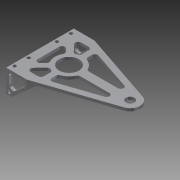
# Autodesk Inventor part: lower bix side plate 3.5
Saved by Autodesk Inventor 2012 (Build 160160000, 160)
## iProperties
Created: 2012-12-28
Part Number: lower bix side plate 3.5
Material: Default
Document SubType Name: Modeling
Designer: Bryce
Density: 1 g/cm^3
Author: Bryce
Autodesk Inventor part; units mm, degrees
ref_plane "YZ Plane" through (0, 0, 0) normal (1, 0, 0) x (0, 1, 0)
ref_plane "XZ Plane" through (0, 0, 0) normal (0, 1, 0) x (-1, 0, 0)
ref_plane "XY Plane" through (0, 0, 0) normal (0, 0, 1) x (1, 0, 0)
sketch "Sketch1" plane through (0, 0, 0) normal (0, 0, 1) x (1, 0, 0)
  line L0 (-34.925, 101.6) -> (34.925, 101.6)
  line L1 (34.925, 101.6) -> (34.925, 68.8594)
  line L2 (-34.925, 68.8594) -> (-34.925, 101.6)
  line L3 (-34.925, 68.8594) -> (-10.5309, -3.5479)
  line L4 (34.925, 68.8594) -> (10.5309, -3.5479)
  arc A0 (-10.5309, -3.5479) -> (10.5309, -3.5479) centre (0, 0) ccw
  circle A1 centre (0, 0) radius 4.7625
  circle A2 centre (0, 68.8594) radius 11.1125
  line L5 (0, 68.8594) -> (-34.925, 68.8594) construction
  line L6 (0, 68.8594) -> (34.925, 68.8594) construction
  line L7 (0, 68.8594) -> (-34.925, 101.6) construction
  line L8 (0, 68.8594) -> (34.925, 101.6) construction
  line L9 (0, 68.8594) -> (0, 0) construction
  line L10 (0, 68.8594) -> (0, 0) construction
  arc A3 (-15.5543, 65.6844) -> (-4.7625, 53.7156) centre (0, 68.8594) ccw
  arc A4 (4.7625, 53.7156) -> (15.5543, 65.6844) centre (0, 68.8594) ccw
  arc A5 (15.5543, 72.0344) -> (13.5191, 77.181) centre (0, 68.8594) ccw
  arc A6 (9.1762, 81.8137) -> (-9.1762, 81.8137) centre (0, 68.8594) ccw
  arc A7 (-13.5191, 77.181) -> (-15.5543, 72.0344) centre (0, 68.8594) ccw
  line L11 (-4.7625, 53.7156) -> (-4.7625, 10.0402)
  line L12 (4.7625, 53.7156) -> (4.7625, 10.0402)
  arc A8 (-4.7625, 10.0402) -> (-7.7188, 7.9942) centre (0, 0) ccw
  arc A9 (7.7188, 7.9942) -> (4.7625, 10.0402) centre (0, 0) ccw
  line L13 (-27.1547, 65.6844) -> (-7.7188, 7.9942)
  line L14 (7.7188, 7.9942) -> (27.1547, 65.6844)
  line L15 (-27.1547, 65.6844) -> (-15.5543, 65.6844)
  line L16 (-28.575, 72.0344) -> (-15.5543, 72.0344)
  line L17 (15.5543, 65.6844) -> (27.1547, 65.6844)
  line L18 (15.5543, 72.0344) -> (28.575, 72.0344)
  line L19 (-28.575, 91.2952) -> (-13.5191, 77.181)
  line L20 (-20.1222, 92.075) -> (-9.1762, 81.8137)
  line L21 (20.1222, 92.075) -> (9.1762, 81.8137)
  line L22 (28.575, 91.2952) -> (13.5191, 77.181)
  line L23 (-28.575, 91.2952) -> (-28.575, 72.0344)
  line L24 (-20.1222, 92.075) -> (20.1222, 92.075)
  line L25 (28.575, 91.2952) -> (28.575, 72.0344)
  arc A10 (4.7625, 18.588) -> (10.9463, 17.5744) centre (7.9375, 18.588) ccw
  arc A11 (-10.9463, 17.5744) -> (-4.7625, 18.588) centre (-7.9375, 18.588) ccw
  point P0 (-31.75, 98.425)
  point P1 (31.75, 98.425)
  point P2 (-15.875, 98.425)
  point P3 (15.875, 98.425)
  dimension "d0" = 69.85
  dimension "d1" = 101.6
  dimension "d2" = 34.925
  dimension "d6" = 18.619
  dimension "d7" = 9.525
  dimension "d8" = 32.7406
  dimension "d9" = 22.225
  dimension "d12" = 15.875
  dimension "d13" = 4.7625
  dimension "d14" = 4.7625
  dimension "d15" = 6.35
  dimension "d16" = 6.35
  dimension "d17" = 3.175
  dimension "d18" = 3.175
  dimension "d19" = 3.175
  dimension "d20" = 3.175
  dimension "d21" = 3.175
  dimension "d22" = 3.175
  dimension "d24" = 3.175
  dimension "d25" = 3.175
  dimension "d26" = 6.35
  dimension "d27" = 9.525
  dimension "d28" = 6.35
  dimension "d32" = 3.175
  dimension "d33" = 3.175
  dimension "d35" = 3.175
  dimension "d36" = 3.175
  dimension "d62" = 19.05
  dimension "d63" = 19.05
  dimension "d69" = 3.175
  dimension "d70" = 18.619
  dimension "d71" = 11.1125
  constraints: 52 end point, 20 point on circle, 13 parallel, 12 centre point, 9 coincident, 7 equal radius, 7 perpendicular, 5 tangent, 4 horizontal alignment, 4 point on line, 1 collinear, 1 horizontal, 1 vertical alignment
  measures "d0" distance between parallel lines of L1 L2
  measures "d1" distance from line of point (0, 0) L0
  measures "d2" distance from line of point (0, 0) L2
  measures "d6" angle of L1 L4
  measures "d7" diameter of A1
  measures "d8" distance from line of L5.start L0
  measures "d9" diameter of A2
  measures "d12" radius of A3
  measures "d13" distance between parallel lines of L9 L11
  measures "d14" distance between parallel lines of L9 L12
  measures "d15" distance between parallel lines of L3 L13
  measures "d16" distance between parallel lines of L4 L14
  measures "d17" distance between parallel lines of L15 L5
  measures "d18" distance between parallel lines of L5 L16
  measures "d19" distance between parallel lines of L17 L6
  measures "d20" distance between parallel lines of L6 L18
  measures "d21" distance between parallel lines of L8 L21
  measures "d22" distance between parallel lines of L8 L22
  measures "d24" distance between parallel lines of L7 L19
  measures "d25" distance between parallel lines of L7 L20
  measures "d26" distance between parallel lines of L23 L2
  measures "d27" distance between parallel lines of L0 L24
  measures "d28" distance between parallel lines of L1 L25
  measures "d32" distance from line of L2 point (-31.75, 98.425)
  measures "d33" distance from line of L0 point (-31.75, 98.425)
  measures "d35" distance from line of L0 point (31.75, 98.425)
  measures "d36" distance from line of L1 point (31.75, 98.425)
  measures "d62" distance from line of L2 point (-15.875, 98.425)
  measures "d63" distance from line of point (15.875, 98.425) L1
  measures "d69" radius of A11
  measures "d70" angle of L3 L2
  measures "d71" radius of A0
extrude "Extrusion1" add sketch "Sketch1" against normal blind 3.175 contours L0 L1 L4 A0 L3 L2 | A3 L11 A11 L13 L15 | L11 A8 L13 A11 | A4 L17 L14 A10 L12 | A10 L14 A9 L12 | A5 L22 L25 L18 | A6 L20 L24 L21 | A7 L16 L23 L19
extrude "Extrusion2" cut sketch "Sketch1" against normal blind 3.175 contours A3 L11 A11 L13 L15 | A4 L17 L14 A10 L12 | A5 L22 L25 L18 | A6 L20 L24 L21 | A7 L16 L23 L19
fillet "Fillet1" radius 3.175 16 edges at (-28.575, 72.0344, -1.5875) (-28.575, 91.2952, -1.5875) (28.575, 91.2952, -1.5875) (28.575, 72.0344, -1.5875) (15.5543, 72.0344, -1.5875) (13.5191, 77.181, -1.5875) (9.1762, 81.8137, -1.5875) (-9.1762, 81.8137, -1.5875) (-13.5191, 77.181, -1.5875) (-15.5543, 72.0344, -1.5875) (15.5543, 65.6844, -1.5875) (27.1547, 65.6844, -1.5875) (4.7625, 53.7156, -1.5875) (-4.7625, 53.7156, -1.5875) (-15.5543, 65.6844, -1.5875) (-27.1547, 65.6844, -1.5875)
hole "Hole1" at (-31.75, 98.425, 0) at (31.75, 98.425, 0) at (-15.875, 98.425, 0) at (15.875, 98.425, 0) direction (0, 0, -1) diameter 3.6576 end through all
sketch "Sketch2" plane through (0, 0, 0) normal (0, 0, 1) x (1, 0, 0)
  line L0 (-20.1222, 92.075) -> (20.1222, 92.075) projected
  circle A0 centre (0, 68.8594) radius 11.1125 projected
  line L1 (34.925, 68.8594) -> (10.5309, -3.5479) projected
  line L2 (34.925, 101.6) -> (34.925, 68.8594) projected
  circle A1 centre (15.875, 98.425) radius 1.8288 projected
  circle A2 centre (-15.875, 98.425) radius 1.8288 projected
  circle A3 centre (-15.875, 98.425) radius 1.8288
  circle A4 centre (15.875, 98.425) radius 1.8288
  line L3 (-10.9463, 17.5744) -> (-25.7435, 61.4957) projected
  line L4 (-34.925, 101.6) -> (34.925, 101.6) projected
  line L5 (-34.925, 68.8594) -> (-38.1, 78.2835)
  line L6 (-38.1, 78.2835) -> (-38.1, 101.6)
  line L7 (-34.925, 101.6) -> (-38.1, 101.6)
  line L8 (34.925, 101.6) -> (38.1, 101.6)
  line L9 (38.1, 101.6) -> (38.1, 78.2835)
  line L10 (38.1, 78.2835) -> (34.925, 68.8594)
  line L11 (-34.925, 101.6) -> (-34.925, 68.8594)
  line L12 (34.925, 101.6) -> (34.925, 68.8594)
  dimension "d53" = 22.225
  dimension "d75" = 3.175
  dimension "d76" = 3.175
  constraints: 16 end point, 4 parallel, 2 centre point, 2 coincident, 2 collinear, 2 concentric, 2 perpendicular
  measures "d53" diameter of A0
  measures "d75" distance of L2.start L8.end
  measures "d76" distance of L4.start L6.end
fillet "Fillet6" radius 3.175 2 edges at (-20.1222, 92.075, -1.5875) (20.1222, 92.075, -1.5875)
extrude "Extrusion7" add sketch "Sketch2" against normal blind 25.4 contours L8 L9 L10 L2 | L5 L6 L7 L11
sketch "Sketch4" plane through (-38.1, 78.2835, 0) normal (-1, 0, 0) x (0, 0, 1)
  line L0 (-25.4, 23.3165) -> (-25.4, 0) projected
  line L1 (0, 23.3165) -> (0, 0) projected
  line L2 (0, 23.3165) -> (-25.4, 23.3165) projected
  circle A0 centre (-22.225, 20.1415) radius 1.7272
  line L3 (-25.4, 16.9665) -> (-3.9692, -7.3236)
  line L4 (-3.175, -9.4241) -> (-3.175, -81.8314) projected
  line L5 (-3.175, -9.4241) -> (-25.4, -9.4241) projected
  line L6 (-25.4, 0) -> (-25.4, -9.4241) projected
  line L7 (0, -81.8314) -> (0, 0) projected
  arc A1 (-3.175, -9.4241) -> (-3.9692, -7.3236) centre (-6.35, -9.4241) ccw
  arc A2 (-20.1746, 15.8429) -> (-17.4625, 20.1415) centre (-22.225, 20.1415) ccw
  line L8 (-20.1746, 15.8429) -> (-3.175, -3.4247)
  line L9 (-3.175, -3.4247) -> (-3.175, 20.1415)
  line L10 (-3.175, 20.1415) -> (-17.4625, 20.1415)
  point P0 (0, -78.2835)
  dimension "d79" = 3.175
  dimension "d80" = 3.175
  dimension "d81" = 3.4544
  dimension "d82" = 3.175
  dimension "d83" = 6.35
  dimension "d84" = 3.175
  dimension "d85" = 4.7625
  dimension "d86" = 3.175
  dimension "d87" = 3.175
  constraints: 8 end point, 4 point on circle, 3 centre point, 2 parallel, 2 tangent, 1 coincident, 1 perpendicular, 1 point on line
  measures "d79" distance from line of L2 A0.centre
  measures "d80" distance from line of L0 A0.centre
  measures "d81" diameter of A0
  measures "d82" radius of A1
  measures "d83" distance from line of L2 L3.start
  measures "d84" distance between parallel lines of L2 L10
  measures "d85" radius of A2
  measures "d86" distance between parallel lines of L3 L8
  measures "d87" distance between parallel lines of L1 L9
extrude "Extrusion8" cut sketch "Sketch4" against normal through all
fillet "Fillet8" radius 3.175 8 edges at (-35.9356, 74.8588, -3.175) (-36.5125, 98.425, -3.175) (-36.5125, 98.425, -17.4625) (-36.5125, 94.1265, -20.1746) (36.5125, 94.1265, -20.1746) (36.5125, 98.425, -17.4625) (36.5125, 98.425, -3.175) (35.9356, 74.8588, -3.175)
body "Solid1"
